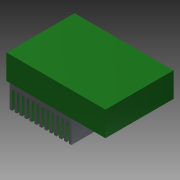
# Autodesk Inventor part: stepper_driver
Saved by Autodesk Inventor 2015 SP1 (Build 190203100, 203)
## iProperties
Created: 2015-04-20
Part Number: stepper_driver
Material: Ogólny
Document SubType Name: Modeling
Designer: Marcin
Density: 1 g/cm^3
Appearance: Gładki - ciemna zieleń leśna
Author: Marcin
Autodesk Inventor part; units mm, degrees
ref_plane "YZ Plane" through (0, 0, 0) normal (1, 0, 0) x (0, 1, 0)
ref_plane "XZ Plane" through (0, 0, 0) normal (0, 1, 0) x (-1, 0, 0)
ref_plane "XY Plane" through (0, 0, 0) normal (0, 0, 1) x (1, 0, 0)
sketch "Szkic1" plane through (0, 0, 0) normal (0, 0, 1) x (1, 0, 0)
  line L0 (-40, -27.5) -> (40, -27.5)
  line L1 (40, -27.5) -> (40, 27.5)
  line L2 (40, 27.5) -> (-40, 27.5)
  line L3 (-40, 27.5) -> (-40, -27.5)
  line L4 (-40, -27.5) -> (40, 27.5) construction
  line L5 (40, -27.5) -> (-40, 27.5) construction
  point P0 (0, 0)
  dimension "d0" = 80
  dimension "d1" = 55
  constraints: 12 end point, 2 midpoint, 2 parallel, 1 horizontal, 1 perpendicular
  measures "d0" distance of L1.end L2.end
  measures "d1" distance of L0.end L1.end
extrude "Wyciągnięcie proste1" add sketch "Szkic1" along normal blind 20
sketch "Szkic2" plane through (0, 0, 0) normal (0, 1, 0) x (-1, 0, 0)
  line L0 (39, 0) -> (-11, 0)
  line L1 (-11, 0) -> (-11, -20)
  line L2 (-11, -20) -> (39, -20)
  line L3 (39, -20) -> (39, 0)
  line L4 (40, 0) -> (40, 20) projected
  line L5 (40, 0) -> (-40, 0) projected
  point P0 (0, 0)
  dimension "d4" = 50
  dimension "d5" = 20
  dimension "d6" = 1
  constraints: 8 end point, 2 parallel, 1 collinear, 1 horizontal, 1 perpendicular
  measures "d4" distance of L2.end L1.end
  measures "d5" distance of L1.end L0.end
  measures "d6" distance between parallel lines of L4 L3
extrude "Wyciągnięcie proste2" add sketch "Szkic2" along normal mid plane 52
sketch "Szkic3" plane through (0, -26, 0) normal (0, -1, 0) x (1, 0, 0)
  line L0 (11, -20) -> (-39, -20) projected
  line L1 (-37, -20) -> (-35, -20)
  line L2 (-35, -20) -> (-35, -5)
  line L3 (-35, -5) -> (-37, -5)
  line L4 (-37, -5) -> (-37, -20)
  line L5 (-39, 0) -> (-39, -20) projected
  line L6 (-33, -20) -> (-31, -20)
  line L7 (-31, -20) -> (-31, -5)
  line L8 (-31, -5) -> (-33, -5)
  line L9 (-33, -5) -> (-33, -20)
  line L10 (-29, -20) -> (-27, -20)
  line L11 (-27, -20) -> (-27, -5)
  line L12 (-27, -5) -> (-29, -5)
  line L13 (-29, -5) -> (-29, -20)
  line L14 (-25, -20) -> (-23, -20)
  line L15 (-23, -20) -> (-23, -5)
  line L16 (-23, -5) -> (-25, -5)
  line L17 (-25, -5) -> (-25, -20)
  line L18 (-21, -20) -> (-19, -20)
  line L19 (-19, -20) -> (-19, -5)
  line L20 (-19, -5) -> (-21, -5)
  line L21 (-21, -5) -> (-21, -20)
  line L22 (-17, -20) -> (-15, -20)
  line L23 (-15, -20) -> (-15, -5)
  line L24 (-15, -5) -> (-17, -5)
  line L25 (-17, -5) -> (-17, -20)
  line L26 (-13, -20) -> (-11, -20)
  line L27 (-11, -20) -> (-11, -5)
  line L28 (-11, -5) -> (-13, -5)
  line L29 (-13, -5) -> (-13, -20)
  line L30 (-9, -20) -> (-7, -20)
  line L31 (-7, -20) -> (-7, -5)
  line L32 (-7, -5) -> (-9, -5)
  line L33 (-9, -5) -> (-9, -20)
  line L34 (-5, -20) -> (-3, -20)
  line L35 (-3, -20) -> (-3, -5)
  line L36 (-3, -5) -> (-5, -5)
  line L37 (-5, -5) -> (-5, -20)
  line L38 (-1, -20) -> (1, -20)
  line L39 (1, -20) -> (1, -5)
  line L40 (1, -5) -> (-1, -5)
  line L41 (-1, -5) -> (-1, -20)
  line L42 (3, -20) -> (5, -20)
  line L43 (5, -20) -> (5, -5)
  line L44 (5, -5) -> (3, -5)
  line L45 (3, -5) -> (3, -20)
  line L46 (7, -20) -> (9, -20)
  line L47 (9, -20) -> (9, -5)
  line L48 (9, -5) -> (7, -5)
  line L49 (7, -5) -> (7, -20)
  point P0 (0, 0)
  dimension "d9" = 2
  dimension "d10" = 15
  dimension "d11" = 2
  dimension "d14" = 4
  constraints: 96 end point, 2 horizontal, 2 parallel, 1 perpendicular, 1 point on line, 88 other
  measures "d9" distance of L2.end L3.end
  measures "d10" distance of L3.end L1.start
  measures "d11" distance between parallel lines of L5 L4
  measures "d14" distance of L1.start L6.start
extrude "Wyciągnięcie proste3" cut sketch "Szkic3" against normal blind 52
